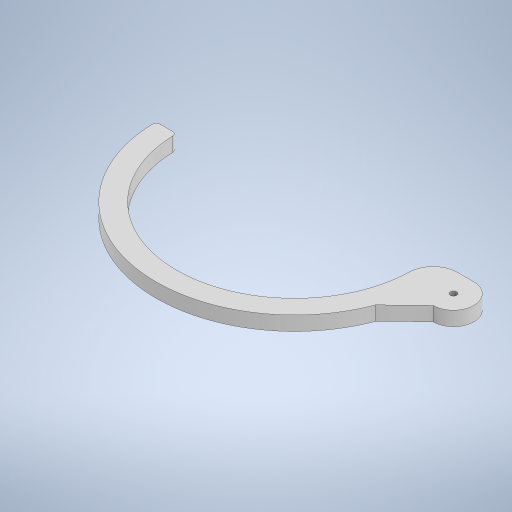
# Autodesk Inventor part: bras_pince_gauche
Saved by Autodesk Inventor 2024.1 (Build 281209000, 209)
## iProperties
Created: 2024-04-06
Part Number: bras_pince_gauche
Material: Générique
Document SubType Name: Modeling
Designer: chass
Density: 1 g/cm^3
Appearance: Par défaut
Author: chass
Autodesk Inventor part; units mm, degrees
ref_plane "YZ Plane" through (0, 0, 0) normal (1, 0, 0) x (0, 1, 0)
ref_plane "XZ Plane" through (0, 0, 0) normal (0, 1, 0) x (-1, 0, 0)
ref_plane "XY Plane" through (0, 0, 0) normal (0, 0, 1) x (1, 0, 0)
sketch "Esquisse1" plane through (0, 0, 0) normal (0, 1, 0) x (-1, 0, 0)
  arc A0 (58, 0) -> (-58, 0) centre (0, 0) ccw
  arc A1 (68, 0) -> (-68, 0) centre (0, 0) ccw
  line L0 (58, 0) -> (68, 0)
  circle A2 centre (-78, 0) radius 10
  circle A3 centre (-78, 0) radius 1.5
  line L1 (-78, 10) -> (-58.201, 10) construction
  line L2 (-78, 10) -> (-63.6239, 24)
  line L3 (-78, -10) -> (-58, -10)
  line L4 (-58, 0) -> (-58, -10)
  dimension "d9" = 58
  dimension "d10" = 68
  dimension "d11" = 20
  dimension "d12" = 20
  dimension "d13" = 3
  constraints: 10 end point, 7 point on circle, 4 centre point, 2 coincident, 2 horizontal, 1 vertical
  measures "d9" radius of A0
  measures "d10" radius of A1
  measures "d11" diameter of A2
  measures "d12" distance of L4.start A2.centre
  measures "d13" diameter of A3
extrude "Extrusion1" add sketch "Esquisse1" along normal blind 7
sketch "Esquisse2" plane through (0, 0, 0) normal (0, -1, 0) x (1, 0, 0)
  circle A0 centre (78, 0) radius 2.6
  point P0 (0, 0)
  dimension "d16" = 5.2
  constraints: 1 centre point
  measures "d16" diameter of A0
extrude "Extrusion2" cut sketch "Esquisse2" against normal blind 4
fillet "Congé1" radius 12 1 edges at (58, 3.5, -10)
fillet "Congé2" radius 2 2 edges at (-68, 3.5, 0) (-58, 3.5, 0)
